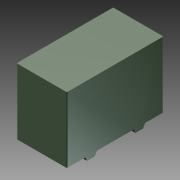
# Autodesk Inventor part: M2T1S03body
Saved by Autodesk Inventor 2011 SP1 (Build 150282100, 282)
## iProperties
Created: 2013-12-24
Part Number: M2T1S03body
Catalog Web Link: www.cadenas.de
Description: M2T Series - Process Sealed Miniature Toggles - Body-
Vendor: NKKSWITCHES
Document SubType Name: Modeling
Designer: PARTuser1
Manufacturer: NKKSWITCHES
Density: 1 g/cm^3
Category: PARTsolutions
Company: NKKSWITCHES
Title: M2T1S03body
Author: Cadenas PARTsolutions
PSOL_IDENT_0: {$CADENAS_DATA\23d-libs\nkkswitches\toggle\m2t\parts\m2t_body.prj},225 {VTYP=3D},{NB=M2T1S03body},{L
PSOL_IDENT_1: INA=M2T1S03body},{NN=M2T Series - Process Sealed Miniature Toggles - Body},{DATE=07.04.2009 06:49:50
PSOL_IDENT_2: },{GEOMDATE=07.04.2009 06:44:00},{VERSION=},{LINEID=10},{LINESUBID=-1},{WBVAR=PLS,ACTU,TRMNLS}  {NB=
PSOL_IDENT_3: M2T1S03body},{LINA=M2T1S03body},{KT=DUMMY},{PN=M2T1S03},{SRS=M2T},{PLS=1},{ACTU=S},{TRMNLS=03},{ALG=
PSOL_IDENT_4: '03','03 - Straight','05','05 - .425\" (10.8mm) Extended PC','06','06 - .750\" (19.05mm) Extended P
PSOL_IDENT_5: C','07','07 - .964\" (24.5mm) Extended PC' }
CNS_NN: M2T Series - Process Sealed Miniature Toggles - Body
CNS_NB: M2T1S03body
CNS_NBSYN: $PN.body
CNS_LINA: M2T1S03body
CNS_PN: M2T1S03
CNS_SRS: M2T
CNS_PLS: 1 - SPDT
CNS_ACTU: S - .500" (12.7mm) Bat Lever
CNS_TRMNLS: 03 - Straight
CNS_ALG: '03','03 - Straight','05','05 - .425" (10.8mm) Extended PC','06','06 - .750" (19.05mm) Extended PC','07','07 - .964" (24.5mm) Extended PC'
SUPPLIER: NKKSWITCHES
ARTICLENO: M2T1S03body
BOMINFO: M2T1S03body
CREATOR: CADENAS GmbH
Autodesk Inventor part; units mm, degrees
sketch "Sketch_1" plane through (0, 0, 0) normal (0, 1, 0) x (-1, 0, 0)
  line L0 (3.302, -6.223) -> (3.302, 6.223)
  arc A0 (3.302, 6.223) -> (3.175, 6.35) centre (3.175, 6.223) ccw
  line L1 (3.175, 6.35) -> (-3.175, 6.35)
  arc A1 (-3.175, 6.35) -> (-3.302, 6.223) centre (-3.175, 6.223) ccw
  line L2 (-3.302, 6.223) -> (-3.302, -6.223)
  arc A2 (-3.302, -6.223) -> (-3.175, -6.35) centre (-3.175, -6.223) ccw
  line L3 (-3.175, -6.35) -> (3.175, -6.35)
  arc A3 (3.175, -6.35) -> (3.302, -6.223) centre (3.175, -6.223) ccw
  constraints: 8 end point, 8 point on circle, 4 centre point
extrude "Extrusion1" add sketch "Sketch_1" along normal mid plane 8.636
sketch "Sketch_2" plane through (3.302, 0, 0) normal (1, 0, 0) x (0, 0, -1)
  line L0 (-3.937, -4.318) -> (-3.683, -4.826)
  line L1 (-3.683, -4.826) -> (-2.667, -4.826)
  line L2 (-2.667, -4.826) -> (-2.413, -4.318)
  line L3 (-2.413, -4.318) -> (-3.937, -4.318)
  constraints: 8 end point
extrude "Extrusion2" add sketch "Sketch_2" against normal blind 0.635
sketch "Sketch_3" plane through (3.302, 0, 0) normal (1, 0, 0) x (0, 0, -1)
  line L0 (2.413, -4.318) -> (2.667, -4.826)
  line L1 (2.667, -4.826) -> (3.683, -4.826)
  line L2 (3.683, -4.826) -> (3.937, -4.318)
  line L3 (3.937, -4.318) -> (2.413, -4.318)
  constraints: 8 end point
extrude "Extrusion3" add sketch "Sketch_3" against normal blind 0.635
sketch "Sketch_4" plane through (-3.302, 0, 0) normal (1, 0, 0) x (0, 0, -1)
  line L0 (-3.937, -4.318) -> (-3.683, -4.826)
  line L1 (-3.683, -4.826) -> (-2.667, -4.826)
  line L2 (-2.667, -4.826) -> (-2.413, -4.318)
  line L3 (-2.413, -4.318) -> (-3.937, -4.318)
  constraints: 8 end point
extrude "Extrusion4" add sketch "Sketch_4" along normal blind 0.635
sketch "Sketch_5" plane through (-3.302, 0, 0) normal (1, 0, 0) x (0, 0, -1)
  line L0 (2.413, -4.318) -> (2.667, -4.826)
  line L1 (2.667, -4.826) -> (3.683, -4.826)
  line L2 (3.683, -4.826) -> (3.937, -4.318)
  line L3 (3.937, -4.318) -> (2.413, -4.318)
  constraints: 8 end point
extrude "Extrusion5" add sketch "Sketch_5" along normal blind 0.635
ref_plane "bushing_XY" through (0, 4.318, 0) normal (0, -1, 0) x (1, 0, 0)
ref_plane "bushing_YZ" through (0, 4.318, 0) normal (1, 0, 0) x (0, 0, 1)
ref_plane "bushing_ZX" through (0, 4.318, 0) normal (0, 0, 1) x (0, -1, 0)
ref_plane "dummy_body_XY" through (0, 0, 0) normal (0, 1, 0) x (1, 0, 0)
ref_plane "dummy_body_YZ" through (0, 0, 0) normal (1, 0, 0) x (0, 0, -1)
ref_plane "dummy_body_ZX" through (0, 0, 0) normal (0, 0, -1) x (0, 1, 0)
ref_plane "terminals_XY" through (0, -4.191, 0) normal (0, 1, 0) x (1, 0, 0)
ref_plane "terminals_YZ" through (0, -4.191, 0) normal (1, 0, 0) x (0, 0, -1)
ref_plane "terminals_ZX" through (0, -4.191, 0) normal (0, 0, -1) x (0, 1, 0)
body "Solid1"
